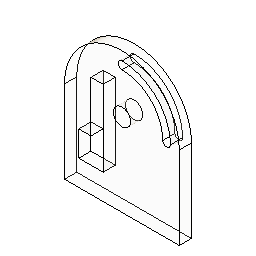
CameraLevel v3 (Autodesk Fusion 360 design; units mm, degrees)
Autodesk Fusion 360 part; units mm, degrees
sketch "Sketch1" plane through (0, 0, 0) normal (0, 1, 0) x (1, 0, 0)
  line L0 (0, 0) -> (-4.8, 0)
  line L1 (-4.8, 0) -> (-4.8, -10)
  line L2 (-4.8, -10) -> (0, -10)
  line L3 (0, -10) -> (0, -30)
  line L4 (0, -30) -> (4.8, -30)
  line L5 (4.8, -30) -> (4.8, 0)
  line L6 (4.8, 0) -> (0, 0)
  line L7 (0, 0) -> (0, -10) construction
  line L8 (-10.4, 10) -> (34.8, 10)
  line L9 (9.8, -25) -> (14.6, -25) construction
  line L10 (14.6, -25) -> (14.6, -20.2) construction
  line L11 (14.6, -20.2) -> (9.8, -20.2) construction
  line L12 (9.8, -20.2) -> (9.8, -25) construction
  line L13 (9.8, -22.6) -> (29.8, -22.6) construction
  line L14 (12.2, -20.2) -> (12.2, -40.2) construction
  circle A0 centre (12.2, -22.6) radius 3.3941
  arc A1 (31.3, -22.6) -> (12.2, -41.7) centre (12.2, -22.6) ccw construction
  arc A2 (12.2, -41.7) -> (31.3, -22.6) centre (12.2, -22.6) ccw
  arc A3 (28.3, -22.6) -> (12.2, -38.7) centre (12.2, -22.6) ccw construction
  arc A4 (12.2, -38.7) -> (28.3, -22.6) centre (12.2, -22.6) ccw
  arc A5 (12.2, -38.7) -> (12.2, -41.7) centre (12.2, -40.2) ccw
  arc A6 (12.2, -41.7) -> (12.2, -38.7) centre (12.2, -40.2) ccw construction
  arc A7 (31.3, -22.6) -> (28.3, -22.6) centre (29.8, -22.6) ccw
  arc A8 (28.3, -22.6) -> (31.3, -22.6) centre (29.8, -22.6) ccw construction
  circle A9 centre (12.2, -40.2) radius 5 construction
  line L15 (-10.4, 10) -> (-10.4, -22.6)
  arc A10 (12.2, -45.2) -> (12.2, -45.2) centre (12.2, -22.6) ccw
  line L16 (34.8, -22.6) -> (34.8, 10)
  line L17 (9.8, -25) -> (4.8, -25) construction
  arc A11 (34.8, -22.6) -> (-10.4, -22.6) centre (12.2, -22.6) ccw construction
  arc A12 (-10.4, -22.6) -> (12.2, -45.2) centre (12.2, -22.6) ccw
  arc A13 (12.2, -45.2) -> (34.8, -22.6) centre (12.2, -22.6) ccw
  point P0 (12.2, -20.2)
  point P1 (9.8, -22.6)
  point P2 (12.2, -22.6)
  dimension "d23" = 4.8
  dimension "d24" = 10
  dimension "d26" = 4.8
  dimension "d27" = 10
  dimension "d31" = 4.8
  dimension "d32" = 4.8
  dimension "d33" = 20
  dimension "d34" = 20
  dimension "d35" = 3
  dimension "d36" = 3
  dimension "d37" = 10
  dimension "d38" = 30
  dimension "d40" = 5
  dimension "d41" = 5
  constraint perpendicular L0 L1
  constraint perpendicular L1 L2
  constraint perpendicular L2 L3
  constraint perpendicular L3 L4
  constraint perpendicular L4 L5
  constraint coincident L0.start L6.end
  constraint perpendicular L2 L7
  constraint parallel L6 L8
  constraint horizontal L9
  constraint vertical L10
  constraint horizontal L11
  constraint vertical L12
  constraint midpoint L11 P0
  constraint midpoint L12 P1
  constraint coincident P1 L13.start
  constraint perpendicular L12 L13
  constraint coincident P0 L14.start
  constraint perpendicular L11 L14
  constraint coincident L13 P2
  constraint coincident L14 P2
  constraint coincident L14.end A5.centre
  constraint coincident L13.end A7.centre
  constraint coincident P2 A0.centre
  constraint coincident L10.end A0
  constraint tangent A3 A7
  constraint concentric A0 A1
  constraint tangent A1 A7
  constraint concentric A1 A2
  constraint coincident L14 A3.end
  constraint coincident L13 A3.start
  constraint concentric A3 A4
  constraint concentric A5 A6
  constraint concentric A7 A8
  constraint concentric A5 A9
  constraint coincident A9 A10.start
  constraint tangent A10 L16
  constraint perpendicular L8 L16
  constraint vertical L15
  constraint collinear L0 L6
  constraint perpendicular L8 L15
  constraint perpendicular L5 L17
  constraint coincident L5 L17.end
  constraint tangent A9 A10
  constraint coincident A10 L16.start
  constraint concentric A0 A11
  constraint tangent A9 A11
  constraint tangent L16 A11
  constraint tangent L15 A11
  constraint concentric A11 A12
  constraint concentric A11 A13
  measures "d23" distance of L0.start L0.end
  measures "d24" distance of L0.end L1.end
  measures "d26" distance of L3.end L4.end
  measures "d27" distance of L6 L8
  measures "d31" distance of L9.start L9.end
  measures "d32" distance of L9.start L11.end
  measures "d33" distance of P1 L13.end
  measures "d34" distance of P0 L14.end
  measures "d35" diameter of A5
  measures "d36" diameter of A7
  measures "d37" diameter of A9
  measures "d38" distance of L4 L6
  measures "d40" distance of L9.start L17.end
  measures "d41" distance of L4 L17
extrude "Extrude1" add sketch "Sketch1" along normal blind 4.8 contours L0 L1 L5 L6 L8 L15 A10 L16 | L1 L2 L3 L4 L5 A10 A12 A13
